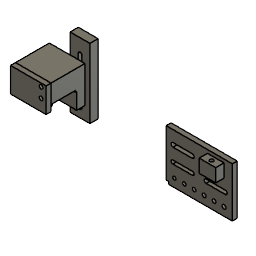
R2_关键配合小样 (Autodesk Fusion 360 design; units mm, degrees)
part number: 2026-09-10-23-08-55-892
part number: 2026-09-10-23-27-46-546
part number: 2026-09-10-23-27-47-376
part number: 2026-09-10-23-27-47-996
part number: 2026-09-10-23-27-48-831
Autodesk Fusion 360 part; units mm, degrees
ref_plane "工作平面1" through (0, 0, 0) normal (0, 0, 1) x (1, 0, 0) in component "CT01_右后承托局部小样"
sketch "草图1" plane through (0, 0, 0) normal (0, 0, 1) x (1, 0, 0) in component "CT01_右后承托局部小样"
  line L0 (-37, 26) -> (6, 26)
  line L1 (6, 26) -> (6, 70)
  line L2 (6, 70) -> (-37, 70)
  line L3 (-37, 70) -> (-37, 26)
  point P0 (-1000, -1000)
  dimension "d14" = 963
  dimension "d15" = 1026
  dimension "d16" = 43
  dimension "d17" = 44
  constraint horizontal L0
  constraint vertical L1
  constraint horizontal L2
  constraint vertical L3
  measures "d14" horizontal distance of L0.start P0
  measures "d15" vertical distance of L0.start P0
  measures "d16" horizontal distance of L0.start L0.end
  measures "d17" vertical distance of L0.end L1.end
extrude "Support_base" add sketch "草图1" along normal blind 10 makes body 1 in component "CT01_右后承托局部小样"
ref_plane "工作平面2" through (0, 0, 10) normal (0, 0, 1) x (1, 0, 0) in component "CT01_右后承托局部小样"
sketch "草图2" plane through (0, 0, 10) normal (0, 0, 1) x (1, 0, 0) in component "CT01_右后承托局部小样"
  line L0 (-37, 47.5) -> (6, 47.5)
  line L1 (6, 47.5) -> (6, 70)
  line L2 (6, 70) -> (-37, 70)
  line L3 (-37, 70) -> (-37, 47.5)
  point P0 (-1000, -1000)
  dimension "d22" = 963
  dimension "d23" = 1047.5
  dimension "d24" = 43
  dimension "d25" = 22.5
  constraint horizontal L0
  constraint vertical L1
  constraint horizontal L2
  constraint vertical L3
  measures "d22" horizontal distance of L0.start P0
  measures "d23" vertical distance of L0.start P0
  measures "d24" horizontal distance of L0.start L0.end
  measures "d25" vertical distance of L0.end L1.end
extrude "Hard_standoff" add sketch "草图2" along normal blind 31 bodies 1 in component "CT01_右后承托局部小样"
ref_plane "工作平面3" through (0, 0, 10) normal (0, 0, 1) x (1, 0, 0) in component "CT01_右后承托局部小样"
sketch "草图3" plane through (0, 0, 10) normal (0, 0, 1) x (1, 0, 0) in component "CT01_右后承托局部小样"
  line L0 (-37, 45.5) -> (6, 45.5)
  line L1 (6, 45.5) -> (6, 47.5)
  line L2 (6, 47.5) -> (-37, 47.5)
  line L3 (-37, 47.5) -> (-37, 45.5)
  point P0 (-1000, -1000)
  dimension "d30" = 963
  dimension "d31" = 1045.5
  dimension "d32" = 43
  dimension "d33" = 2
  constraint horizontal L0
  constraint vertical L1
  constraint horizontal L2
  constraint vertical L3
  measures "d30" horizontal distance of L0.start P0
  measures "d31" vertical distance of L0.start P0
  measures "d32" horizontal distance of L0.start L0.end
  measures "d33" vertical distance of L0.end L1.end
extrude "Lower_Y_stop" add sketch "草图3" along normal blind 1.5 bodies 1 in component "CT01_右后承托局部小样"
ref_plane "工作平面4" through (0, 0, 39.5) normal (0, 0, 1) x (1, 0, 0) in component "CT01_右后承托局部小样"
sketch "草图4" plane through (0, 0, 39.5) normal (0, 0, 1) x (1, 0, 0) in component "CT01_右后承托局部小样"
  line L0 (-37, 45.5) -> (6, 45.5)
  line L1 (6, 45.5) -> (6, 47.5)
  line L2 (6, 47.5) -> (-37, 47.5)
  line L3 (-37, 47.5) -> (-37, 45.5)
  point P0 (-1000, -1000)
  dimension "d38" = 963
  dimension "d39" = 1045.5
  dimension "d40" = 43
  dimension "d41" = 2
  constraint horizontal L0
  constraint vertical L1
  constraint horizontal L2
  constraint vertical L3
  measures "d38" horizontal distance of L0.start P0
  measures "d39" vertical distance of L0.start P0
  measures "d40" horizontal distance of L0.start L0.end
  measures "d41" vertical distance of L0.end L1.end
extrude "Upper_Y_stop" add sketch "草图4" along normal blind 1.5 bodies 1 in component "CT01_右后承托局部小样"
ref_plane "工作平面5" through (0, 0, -1) normal (0, 0, 1) x (1, 0, 0) in component "CT01_右后承托局部小样"
sketch "草图5" plane through (0, 0, -1) normal (0, 0, 1) x (1, 0, 0) in component "CT01_右后承托局部小样"
  circle A0 centre (0, 54) radius 2.25
  point P0 (-1000, -1000)
  dimension "d46" = 1000
  dimension "d47" = 1054
  dimension "d48" = 4.5
  measures "d46" horizontal distance of A0.centre P0
  measures "d47" vertical distance of A0.centre P0
  measures "d48" diameter of A0
extrude "Two_through_bolts_1" cut sketch "草图5" along normal blind 43 bodies 1 in component "CT01_右后承托局部小样"
ref_plane "工作平面6" through (0, 0, -1) normal (0, 0, 1) x (1, 0, 0) in component "CT01_右后承托局部小样"
sketch "草图6" plane through (0, 0, -1) normal (0, 0, 1) x (1, 0, 0) in component "CT01_右后承托局部小样"
  circle A0 centre (0, 66) radius 2.25
  point P0 (-1000, -1000)
  dimension "d53" = 1000
  dimension "d54" = 1066
  dimension "d55" = 4.5
  measures "d53" horizontal distance of A0.centre P0
  measures "d54" vertical distance of A0.centre P0
  measures "d55" diameter of A0
extrude "Two_through_bolts_2" cut sketch "草图6" along normal blind 43 bodies 1 in component "CT01_右后承托局部小样"
ref_plane "工作平面1" through (0, 0, 41) normal (0, 0, 1) x (1, 0, 0) in component "CT02_右后防脱及X止挡局部小样"
sketch "草图1 (2)" plane through (0, 0, 41) normal (0, 0, 1) x (1, 0, 0) in component "CT02_右后防脱及X止挡局部小样"
  line L0 (-37, 40) -> (6, 40)
  line L1 (6, 40) -> (6, 70)
  line L2 (6, 70) -> (-37, 70)
  line L3 (-37, 70) -> (-37, 40)
  point P0 (-1000, -1000)
  dimension "d60" = 963
  dimension "d61" = 1040
  dimension "d62" = 43
  dimension "d63" = 30
  constraint horizontal L0
  constraint vertical L1
  constraint horizontal L2
  constraint vertical L3
  measures "d60" horizontal distance of L0.start P0
  measures "d61" vertical distance of L0.start P0
  measures "d62" horizontal distance of L0.start L0.end
  measures "d63" vertical distance of L0.end L1.end
extrude "Retainer" add sketch "草图1 (2)" along normal blind 6 separate body makes body 2 in component "CT02_右后防脱及X止挡局部小样"
ref_plane "工作平面2" through (0, 0, 39.5) normal (0, 0, 1) x (1, 0, 0) in component "CT02_右后防脱及X止挡局部小样"
sketch "草图2 (2)" plane through (0, 0, 39.5) normal (0, 0, 1) x (1, 0, 0) in component "CT02_右后防脱及X止挡局部小样"
  line L0 (-19.5, 40) -> (-15.5, 40)
  line L1 (-15.5, 40) -> (-15.5, 44.75)
  line L2 (-15.5, 44.75) -> (-19.5, 44.75)
  line L3 (-19.5, 44.75) -> (-19.5, 40)
  point P0 (-1000, -1000)
  dimension "d68" = 980.5
  dimension "d69" = 1040
  dimension "d70" = 4
  dimension "d71" = 4.75
  constraint horizontal L0
  constraint vertical L1
  constraint horizontal L2
  constraint vertical L3
  measures "d68" horizontal distance of L0.start P0
  measures "d69" vertical distance of L0.start P0
  measures "d70" horizontal distance of L0.start L0.end
  measures "d71" vertical distance of L0.end L1.end
extrude "Upper_X_stop" add sketch "草图2 (2)" along normal blind 1.5 bodies 2 in component "CT02_右后防脱及X止挡局部小样"
ref_plane "工作平面3" through (0, 0, 40) normal (0, 0, 1) x (1, 0, 0) in component "CT02_右后防脱及X止挡局部小样"
sketch "草图3 (2)" plane through (0, 0, 40) normal (0, 0, 1) x (1, 0, 0) in component "CT02_右后防脱及X止挡局部小样"
  circle A0 centre (0, 54) radius 2.25
  point P0 (-1000, -1000)
  dimension "d76" = 1000
  dimension "d77" = 1054
  dimension "d78" = 4.5
  measures "d76" horizontal distance of A0.centre P0
  measures "d77" vertical distance of A0.centre P0
  measures "d78" diameter of A0
extrude "Two_through_bolts_1'" cut sketch "草图3 (2)" along normal blind 8 bodies 2 in component "CT02_右后防脱及X止挡局部小样"
ref_plane "工作平面4" through (0, 0, 40) normal (0, 0, 1) x (1, 0, 0) in component "CT02_右后防脱及X止挡局部小样"
sketch "草图4 (2)" plane through (0, 0, 40) normal (0, 0, 1) x (1, 0, 0) in component "CT02_右后防脱及X止挡局部小样"
  circle A0 centre (0, 66) radius 2.25
  point P0 (-1000, -1000)
  dimension "d83" = 1000
  dimension "d84" = 1066
  dimension "d85" = 4.5
  measures "d83" horizontal distance of A0.centre P0
  measures "d84" vertical distance of A0.centre P0
  measures "d85" diameter of A0
extrude "Two_through_bolts_2'" cut sketch "草图4 (2)" along normal blind 8 bodies 2 in component "CT02_右后防脱及X止挡局部小样"
ref_plane "工作平面1" through (0, 0, -10) normal (0, 0, 1) x (1, 0, 0) in component "CT03_托臂槽段试装垫座"
sketch "草图1 (3)" plane through (0, 0, -10) normal (0, 0, 1) x (1, 0, 0) in component "CT03_托臂槽段试装垫座"
  line L0 (-12, 10) -> (12, 10)
  line L1 (12, 10) -> (12, 94)
  line L2 (12, 94) -> (-12, 94)
  line L3 (-12, 94) -> (-12, 10)
  point P0 (-1000, -1000)
  dimension "d90" = 988
  dimension "d91" = 1010
  dimension "d92" = 24
  dimension "d93" = 84
  constraint horizontal L0
  constraint vertical L1
  constraint horizontal L2
  constraint vertical L3
  measures "d90" horizontal distance of L0.start P0
  measures "d91" vertical distance of L0.start P0
  measures "d92" horizontal distance of L0.start L0.end
  measures "d93" vertical distance of L0.end L1.end
extrude "Arm_segment" add sketch "草图1 (3)" along normal blind 10 separate body makes body 3 in component "CT03_托臂槽段试装垫座"
ref_plane "工作平面2" through (0, 0, -11) normal (0, 0, 1) x (1, 0, 0) in component "CT03_托臂槽段试装垫座"
sketch "草图2 (3)" plane through (0, 0, -11) normal (0, 0, 1) x (1, 0, 0) in component "CT03_托臂槽段试装垫座"
  line L0 (-2.25, 21.25) -> (2.25, 21.25)
  line L1 (2.25, 21.25) -> (2.25, 76.75)
  line L2 (2.25, 76.75) -> (-2.25, 76.75)
  line L3 (-2.25, 76.75) -> (-2.25, 21.25)
  point P0 (-1000, -1000)
  dimension "d98" = 997.75
  dimension "d99" = 1021.25
  dimension "d100" = 4.5
  dimension "d101" = 55.5
  constraint horizontal L0
  constraint vertical L1
  constraint horizontal L2
  constraint vertical L3
  measures "d98" horizontal distance of L0.start P0
  measures "d99" vertical distance of L0.start P0
  measures "d100" horizontal distance of L0.start L0.end
  measures "d101" vertical distance of L0.end L1.end
extrude "Pad_mount_slot_0_middle" cut sketch "草图2 (3)" along normal blind 12 bodies 3 in component "CT03_托臂槽段试装垫座"
ref_plane "工作平面3" through (0, 0, -11) normal (0, 0, 1) x (1, 0, 0) in component "CT03_托臂槽段试装垫座"
sketch "草图3 (3)" plane through (0, 0, -11) normal (0, 0, 1) x (1, 0, 0) in component "CT03_托臂槽段试装垫座"
  circle A0 centre (0, 21.25) radius 2.25
  point P0 (-1000, -1000)
  dimension "d106" = 1000
  dimension "d107" = 1021.25
  dimension "d108" = 4.5
  measures "d106" horizontal distance of A0.centre P0
  measures "d107" vertical distance of A0.centre P0
  measures "d108" diameter of A0
extrude "Pad_mount_slot_0_ends_1" cut sketch "草图3 (3)" along normal blind 12 bodies 3 in component "CT03_托臂槽段试装垫座"
ref_plane "工作平面4" through (0, 0, -11) normal (0, 0, 1) x (1, 0, 0) in component "CT03_托臂槽段试装垫座"
sketch "草图4 (3)" plane through (0, 0, -11) normal (0, 0, 1) x (1, 0, 0) in component "CT03_托臂槽段试装垫座"
  circle A0 centre (0, 76.75) radius 2.25
  point P0 (-1000, -1000)
  dimension "d113" = 1000
  dimension "d114" = 1076.75
  dimension "d115" = 4.5
  measures "d113" horizontal distance of A0.centre P0
  measures "d114" vertical distance of A0.centre P0
  measures "d115" diameter of A0
extrude "Pad_mount_slot_0_ends_2" cut sketch "草图4 (3)" along normal blind 12 bodies 3 in component "CT03_托臂槽段试装垫座"
ref_plane "工作平面1" through (0, 0, 0) normal (0, 0, 1) x (1, 0, 0) in component "HT01_孔槽及横孔试片"
sketch "草图1 (4)" plane through (0, 0, 0) normal (0, 0, 1) x (1, 0, 0) in component "HT01_孔槽及横孔试片"
  line L0 (0, 0) -> (80, 0)
  line L1 (80, 0) -> (80, 60)
  line L2 (80, 60) -> (0, 60)
  line L3 (0, 60) -> (0, 0)
  point P0 (-1000, -1000)
  dimension "d120" = 1000
  dimension "d121" = 1000
  dimension "d122" = 80
  dimension "d123" = 60
  constraint horizontal L0
  constraint vertical L1
  constraint horizontal L2
  constraint vertical L3
  measures "d120" horizontal distance of L0.start P0
  measures "d121" vertical distance of L0.start P0
  measures "d122" horizontal distance of L0.start L0.end
  measures "d123" vertical distance of L0.end L1.end
extrude "Base" add sketch "草图1 (4)" along normal blind 6 separate body makes body 4 in component "HT01_孔槽及横孔试片"
ref_plane "工作平面2" through (0, 0, -1) normal (0, 0, 1) x (1, 0, 0) in component "HT01_孔槽及横孔试片"
sketch "草图2 (4)" plane through (0, 0, -1) normal (0, 0, 1) x (1, 0, 0) in component "HT01_孔槽及横孔试片"
  circle A0 centre (10, 10) radius 2
  point P0 (-1000, -1000)
  dimension "d128" = 1010
  dimension "d129" = 1010
  dimension "d130" = 4
  measures "d128" horizontal distance of A0.centre P0
  measures "d129" vertical distance of A0.centre P0
  measures "d130" diameter of A0
extrude "Vertical_4_1" cut sketch "草图2 (4)" along normal blind 8 bodies 4 in component "HT01_孔槽及横孔试片"
ref_plane "工作平面3" through (0, 0, -1) normal (0, 0, 1) x (1, 0, 0) in component "HT01_孔槽及横孔试片"
sketch "草图3 (4)" plane through (0, 0, -1) normal (0, 0, 1) x (1, 0, 0) in component "HT01_孔槽及横孔试片"
  circle A0 centre (22, 10) radius 2.1
  point P0 (-1000, -1000)
  dimension "d135" = 1022
  dimension "d136" = 1010
  dimension "d137" = 4.2
  measures "d135" horizontal distance of A0.centre P0
  measures "d136" vertical distance of A0.centre P0
  measures "d137" diameter of A0
extrude "Vertical_4.2_1" cut sketch "草图3 (4)" along normal blind 8 bodies 4 in component "HT01_孔槽及横孔试片"
ref_plane "工作平面4" through (0, 0, -1) normal (0, 0, 1) x (1, 0, 0) in component "HT01_孔槽及横孔试片"
sketch "草图4 (4)" plane through (0, 0, -1) normal (0, 0, 1) x (1, 0, 0) in component "HT01_孔槽及横孔试片"
  circle A0 centre (34, 10) radius 2.2
  point P0 (-1000, -1000)
  dimension "d142" = 1034
  dimension "d143" = 1010
  dimension "d144" = 4.4
  measures "d142" horizontal distance of A0.centre P0
  measures "d143" vertical distance of A0.centre P0
  measures "d144" diameter of A0
extrude "Vertical_4.4_1" cut sketch "草图4 (4)" along normal blind 8 bodies 4 in component "HT01_孔槽及横孔试片"
ref_plane "工作平面5" through (0, 0, -1) normal (0, 0, 1) x (1, 0, 0) in component "HT01_孔槽及横孔试片"
sketch "草图5 (2)" plane through (0, 0, -1) normal (0, 0, 1) x (1, 0, 0) in component "HT01_孔槽及横孔试片"
  circle A0 centre (46, 10) radius 2.25
  point P0 (-1000, -1000)
  dimension "d149" = 1046
  dimension "d150" = 1010
  dimension "d151" = 4.5
  measures "d149" horizontal distance of A0.centre P0
  measures "d150" vertical distance of A0.centre P0
  measures "d151" diameter of A0
extrude "Vertical_4.5_1" cut sketch "草图5 (2)" along normal blind 8 bodies 4 in component "HT01_孔槽及横孔试片"
ref_plane "工作平面6" through (0, 0, -1) normal (0, 0, 1) x (1, 0, 0) in component "HT01_孔槽及横孔试片"
sketch "草图6 (2)" plane through (0, 0, -1) normal (0, 0, 1) x (1, 0, 0) in component "HT01_孔槽及横孔试片"
  circle A0 centre (58, 10) radius 2.3
  point P0 (-1000, -1000)
  dimension "d156" = 1058
  dimension "d157" = 1010
  dimension "d158" = 4.6
  measures "d156" horizontal distance of A0.centre P0
  measures "d157" vertical distance of A0.centre P0
  measures "d158" diameter of A0
extrude "Vertical_4.6_1" cut sketch "草图6 (2)" along normal blind 8 bodies 4 in component "HT01_孔槽及横孔试片"
ref_plane "工作平面7" through (0, 0, -1) normal (0, 0, 1) x (1, 0, 0) in component "HT01_孔槽及横孔试片"
sketch "草图7" plane through (0, 0, -1) normal (0, 0, 1) x (1, 0, 0) in component "HT01_孔槽及横孔试片"
  circle A0 centre (70, 10) radius 2.4
  point P0 (-1000, -1000)
  dimension "d163" = 1070
  dimension "d164" = 1010
  dimension "d165" = 4.8
  measures "d163" horizontal distance of A0.centre P0
  measures "d164" vertical distance of A0.centre P0
  measures "d165" diameter of A0
extrude "Vertical_4.8_1" cut sketch "草图7" along normal blind 8 bodies 4 in component "HT01_孔槽及横孔试片"
ref_plane "工作平面8" through (0, 0, -1) normal (0, 0, 1) x (1, 0, 0) in component "HT01_孔槽及横孔试片"
sketch "草图8" plane through (0, 0, -1) normal (0, 0, 1) x (1, 0, 0) in component "HT01_孔槽及横孔试片"
  line L0 (8.1, 23.9) -> (31.9, 23.9)
  line L1 (31.9, 23.9) -> (31.9, 28.1)
  line L2 (31.9, 28.1) -> (8.1, 28.1)
  line L3 (8.1, 28.1) -> (8.1, 23.9)
  point P0 (-1000, -1000)
  dimension "d170" = 1008.1
  dimension "d171" = 1023.9
  dimension "d172" = 23.8
  dimension "d173" = 4.2
  constraint horizontal L0
  constraint vertical L1
  constraint horizontal L2
  constraint vertical L3
  measures "d170" horizontal distance of L0.start P0
  measures "d171" vertical distance of L0.start P0
  measures "d172" horizontal distance of L0.start L0.end
  measures "d173" vertical distance of L0.end L1.end
extrude "Slot_4.2_0_middle" cut sketch "草图8" along normal blind 8 bodies 4 in component "HT01_孔槽及横孔试片"
ref_plane "工作平面9" through (0, 0, -1) normal (0, 0, 1) x (1, 0, 0) in component "HT01_孔槽及横孔试片"
sketch "草图9" plane through (0, 0, -1) normal (0, 0, 1) x (1, 0, 0) in component "HT01_孔槽及横孔试片"
  circle A0 centre (8.1, 26) radius 2.1
  point P0 (-1000, -1000)
  dimension "d178" = 1008.1
  dimension "d179" = 1026
  dimension "d180" = 4.2
  measures "d178" horizontal distance of A0.centre P0
  measures "d179" vertical distance of A0.centre P0
  measures "d180" diameter of A0
extrude "Slot_4.2_0_ends_1" cut sketch "草图9" along normal blind 8 bodies 4 in component "HT01_孔槽及横孔试片"
ref_plane "工作平面10" through (0, 0, -1) normal (0, 0, 1) x (1, 0, 0) in component "HT01_孔槽及横孔试片"
sketch "草图10" plane through (0, 0, -1) normal (0, 0, 1) x (1, 0, 0) in component "HT01_孔槽及横孔试片"
  circle A0 centre (31.9, 26) radius 2.1
  point P0 (-1000, -1000)
  dimension "d185" = 1031.9
  dimension "d186" = 1026
  dimension "d187" = 4.2
  measures "d185" horizontal distance of A0.centre P0
  measures "d186" vertical distance of A0.centre P0
  measures "d187" diameter of A0
extrude "Slot_4.2_0_ends_2" cut sketch "草图10" along normal blind 8 bodies 4 in component "HT01_孔槽及横孔试片"
ref_plane "工作平面11" through (0, 0, -1) normal (0, 0, 1) x (1, 0, 0) in component "HT01_孔槽及横孔试片"
sketch "草图11" plane through (0, 0, -1) normal (0, 0, 1) x (1, 0, 0) in component "HT01_孔槽及横孔试片"
  line L0 (48.25, 23.75) -> (71.75, 23.75)
  line L1 (71.75, 23.75) -> (71.75, 28.25)
  line L2 (71.75, 28.25) -> (48.25, 28.25)
  line L3 (48.25, 28.25) -> (48.25, 23.75)
  point P0 (-1000, -1000)
  dimension "d192" = 1048.25
  dimension "d193" = 1023.75
  dimension "d194" = 23.5
  dimension "d195" = 4.5
  constraint horizontal L0
  constraint vertical L1
  constraint horizontal L2
  constraint vertical L3
  measures "d192" horizontal distance of L0.start P0
  measures "d193" vertical distance of L0.start P0
  measures "d194" horizontal distance of L0.start L0.end
  measures "d195" vertical distance of L0.end L1.end
extrude "Slot_4.5_0_middle" cut sketch "草图11" along normal blind 8 bodies 4 in component "HT01_孔槽及横孔试片"
ref_plane "工作平面12" through (0, 0, -1) normal (0, 0, 1) x (1, 0, 0) in component "HT01_孔槽及横孔试片"
sketch "草图12" plane through (0, 0, -1) normal (0, 0, 1) x (1, 0, 0) in component "HT01_孔槽及横孔试片"
  circle A0 centre (48.25, 26) radius 2.25
  point P0 (-1000, -1000)
  dimension "d200" = 1048.25
  dimension "d201" = 1026
  dimension "d202" = 4.5
  measures "d200" horizontal distance of A0.centre P0
  measures "d201" vertical distance of A0.centre P0
  measures "d202" diameter of A0
extrude "Slot_4.5_0_ends_1" cut sketch "草图12" along normal blind 8 bodies 4 in component "HT01_孔槽及横孔试片"
ref_plane "工作平面13" through (0, 0, -1) normal (0, 0, 1) x (1, 0, 0) in component "HT01_孔槽及横孔试片"
sketch "草图13" plane through (0, 0, -1) normal (0, 0, 1) x (1, 0, 0) in component "HT01_孔槽及横孔试片"
  circle A0 centre (71.75, 26) radius 2.25
  point P0 (-1000, -1000)
  dimension "d207" = 1071.75
  dimension "d208" = 1026
  dimension "d209" = 4.5
  measures "d207" horizontal distance of A0.centre P0
  measures "d208" vertical distance of A0.centre P0
  measures "d209" diameter of A0
extrude "Slot_4.5_0_ends_2" cut sketch "草图13" along normal blind 8 bodies 4 in component "HT01_孔槽及横孔试片"
ref_plane "工作平面14" through (0, 0, -1) normal (0, 0, 1) x (1, 0, 0) in component "HT01_孔槽及横孔试片"
sketch "草图14" plane through (0, 0, -1) normal (0, 0, 1) x (1, 0, 0) in component "HT01_孔槽及横孔试片"
  line L0 (8.4, 41.6) -> (31.6, 41.6)
  line L1 (31.6, 41.6) -> (31.6, 46.4)
  line L2 (31.6, 46.4) -> (8.4, 46.4)
  line L3 (8.4, 46.4) -> (8.4, 41.6)
  point P0 (-1000, -1000)
  dimension "d214" = 1008.4
  dimension "d215" = 1041.6
  dimension "d216" = 23.2
  dimension "d217" = 4.8
  constraint horizontal L0
  constraint vertical L1
  constraint horizontal L2
  constraint vertical L3
  measures "d214" horizontal distance of L0.start P0
  measures "d215" vertical distance of L0.start P0
  measures "d216" horizontal distance of L0.start L0.end
  measures "d217" vertical distance of L0.end L1.end
extrude "Slot_4.8_0_middle" cut sketch "草图14" along normal blind 8 bodies 4 in component "HT01_孔槽及横孔试片"
ref_plane "工作平面15" through (0, 0, -1) normal (0, 0, 1) x (1, 0, 0) in component "HT01_孔槽及横孔试片"
sketch "草图15" plane through (0, 0, -1) normal (0, 0, 1) x (1, 0, 0) in component "HT01_孔槽及横孔试片"
  circle A0 centre (8.4, 44) radius 2.4
  point P0 (-1000, -1000)
  dimension "d222" = 1008.4
  dimension "d223" = 1044
  dimension "d224" = 4.8
  measures "d222" horizontal distance of A0.centre P0
  measures "d223" vertical distance of A0.centre P0
  measures "d224" diameter of A0
extrude "Slot_4.8_0_ends_1" cut sketch "草图15" along normal blind 8 bodies 4 in component "HT01_孔槽及横孔试片"
ref_plane "工作平面16" through (0, 0, -1) normal (0, 0, 1) x (1, 0, 0) in component "HT01_孔槽及横孔试片"
sketch "草图16" plane through (0, 0, -1) normal (0, 0, 1) x (1, 0, 0) in component "HT01_孔槽及横孔试片"
  circle A0 centre (31.6, 44) radius 2.4
  point P0 (-1000, -1000)
  dimension "d229" = 1031.6
  dimension "d230" = 1044
  dimension "d231" = 4.8
  measures "d229" horizontal distance of A0.centre P0
  measures "d230" vertical distance of A0.centre P0
  measures "d231" diameter of A0
extrude "Slot_4.8_0_ends_2" cut sketch "草图16" along normal blind 8 bodies 4 in component "HT01_孔槽及横孔试片"
ref_plane "工作平面17" through (0, 0, 6) normal (0, 0, 1) x (1, 0, 0) in component "HT01_孔槽及横孔试片"
sketch "草图17" plane through (0, 0, 6) normal (0, 0, 1) x (1, 0, 0) in component "HT01_孔槽及横孔试片"
  line L0 (50, 40) -> (70, 40)
  line L1 (70, 40) -> (70, 56)
  line L2 (70, 56) -> (50, 56)
  line L3 (50, 56) -> (50, 40)
  point P0 (-1000, -1000)
  dimension "d236" = 1050
  dimension "d237" = 1040
  dimension "d238" = 20
  dimension "d239" = 16
  constraint horizontal L0
  constraint vertical L1
  constraint horizontal L2
  constraint vertical L3
  measures "d236" horizontal distance of L0.start P0
  measures "d237" vertical distance of L0.start P0
  measures "d238" horizontal distance of L0.start L0.end
  measures "d239" vertical distance of L0.end L1.end
extrude "Horizontal_hole_boss" add sketch "草图17" along normal blind 10 bodies 4 in component "HT01_孔槽及横孔试片"
ref_plane "工作平面18" through (0, 39, 0) normal (0, 1, 0) x (0, 0, 1) in component "HT01_孔槽及横孔试片"
sketch "草图18" plane through (0, 39, 0) normal (0, 1, 0) x (1, 0, 0) in component "HT01_孔槽及横孔试片"
  circle A0 centre (60, -11) radius 2.25
  point P0 (-1000, -1000)
  dimension "d244" = 1060
  dimension "d245" = 989
  dimension "d246" = 4.5
  measures "d244" horizontal distance of A0.centre P0
  measures "d245" vertical distance of A0.centre P0
  measures "d246" diameter of A0
extrude "Horizontal_M4_1" cut sketch "草图18" along normal blind 18 bodies 4 in component "HT01_孔槽及横孔试片"
ref_plane "工作平面19" through (0, 0, -1) normal (0, 0, 1) x (1, 0, 0) in component "HT01_孔槽及横孔试片"
sketch "草图19" plane through (0, 0, -1) normal (0, 0, 1) x (1, 0, 0) in component "HT01_孔槽及横孔试片"
  line L0 (0, 0) -> (3, 0)
  line L1 (3, 0) -> (3, 3)
  line L2 (3, 3) -> (0, 3)
  line L3 (0, 3) -> (0, 0)
  point P0 (-1000, -1000)
  dimension "d251" = 1000
  dimension "d252" = 1000
  dimension "d253" = 3
  dimension "d254" = 3
  constraint horizontal L0
  constraint vertical L1
  constraint horizontal L2
  constraint vertical L3
  measures "d251" horizontal distance of L0.start P0
  measures "d252" vertical distance of L0.start P0
  measures "d253" horizontal distance of L0.start L0.end
  measures "d254" vertical distance of L0.end L1.end
extrude "Origin_notch" cut sketch "草图19" along normal blind 8 bodies 4 in component "HT01_孔槽及横孔试片"
component "CT01_右后承托局部小样" placed x (1, 0, 0) y (0, 1, 0) z (0, 0, 1) at (0, 0, 0)
component "CT02_右后防脱及X止挡局部小样" placed x (1, 0, 0) y (0, 1, 0) z (0, 0, 1) at (0, 0, 0)
component "CT03_托臂槽段试装垫座" placed x (1, 0, 0) y (0, 1, 0) z (0, 0, 1) at (0, 0, 0)
component "HT01_孔槽及横孔试片" placed x (1, 0, 0) y (0, 1, 0) z (0, 0, 1) at (110, 0, 0)
equation "pad_w = 74 mm" comment "TEST_COUPON_ASSUMED_VERIFY_WITH_REAL_PARTS"
equation "coupon_w = 43 mm" comment "TEST_COUPON_ASSUMED_VERIFY_WITH_REAL_PARTS"
equation "board_w = 90 mm" comment "TEST_COUPON_ASSUMED_VERIFY_WITH_REAL_PARTS"
equation "pad_t = 10 mm" comment "TEST_COUPON_ASSUMED_VERIFY_WITH_REAL_PARTS"
equation "soft_t = 0.5 mm" comment "TEST_COUPON_ASSUMED_VERIFY_WITH_REAL_PARTS"
equation "stack_h = 30 mm" comment "TEST_COUPON_ASSUMED_VERIFY_WITH_REAL_PARTS"
equation "retainer_gap = 0.5 mm" comment "TEST_COUPON_ASSUMED_VERIFY_WITH_REAL_PARTS"
equation "lateral_gap = 1 mm" comment "TEST_COUPON_ASSUMED_VERIFY_WITH_REAL_PARTS"
equation "acrylic_t = 1 mm" comment "TEST_COUPON_ASSUMED_VERIFY_WITH_REAL_PARTS"
equation "slot_d = 4.5 mm" comment "TEST_COUPON_ASSUMED_VERIFY_WITH_REAL_PARTS"
equation "support_depth = 19 mm" comment "TEST_COUPON_ASSUMED_VERIFY_WITH_REAL_PARTS"
equation "d14 = 1000 mm + ( -pad_w / 2 )"
equation "d15 = 1000 mm + ( board_w / 2 - support_depth )"
equation "d16 = coupon_w"
equation "d18 = pad_t"
equation "d20 = pad_t"
equation "d22 = 1000 mm + ( -pad_w / 2 )"
equation "d23 = 1000 mm + ( board_w / 2 + lateral_gap / 2 + 2 mm )"
equation "d24 = coupon_w"
equation "d25 = 25 mm - lateral_gap / 2 - 2 mm"
equation "d26 = soft_t + stack_h + retainer_gap"
equation "d28 = pad_t"
equation "d30 = 1000 mm + ( -pad_w / 2 )"
equation "d31 = 1000 mm + ( board_w / 2 + lateral_gap / 2 )"
equation "d32 = coupon_w"
equation "d34 = soft_t + acrylic_t"
equation "d36 = pad_t + soft_t + stack_h - acrylic_t"
equation "d38 = 1000 mm + ( -pad_w / 2 )"
equation "d39 = 1000 mm + ( board_w / 2 + lateral_gap / 2 )"
equation "d40 = coupon_w"
equation "d42 = acrylic_t + retainer_gap"
equation "d46 = 1000 mm + ( 0 mm )"
equation "d47 = 1000 mm + ( 54 mm )"
equation "d48 = slot_d"
equation "d49 = pad_t + soft_t + stack_h + retainer_gap + 2 mm"
equation "d53 = 1000 mm + ( 0 mm )"
equation "d54 = 1000 mm + ( 66 mm )"
equation "d55 = slot_d"
equation "d56 = pad_t + soft_t + stack_h + retainer_gap + 2 mm"
equation "d58 = pad_t + soft_t + stack_h + retainer_gap"
equation "d60 = 1000 mm + ( -pad_w / 2 )"
equation "d61 = 1000 mm + ( 40 mm )"
equation "d62 = coupon_w"
equation "d66 = pad_t + soft_t + stack_h - acrylic_t"
equation "d68 = 1000 mm + ( -20 mm + lateral_gap / 2 )"
equation "d69 = 1000 mm + ( 40 mm )"
equation "d72 = acrylic_t + retainer_gap"
equation "d74 = pad_t + soft_t + stack_h + retainer_gap - 1 mm"
equation "d76 = 1000 mm + ( 0 mm )"
equation "d77 = 1000 mm + ( 54 mm )"
equation "d78 = slot_d"
equation "d81 = pad_t + soft_t + stack_h + retainer_gap - 1 mm"
equation "d83 = 1000 mm + ( 0 mm )"
equation "d84 = 1000 mm + ( 66 mm )"
equation "d85 = slot_d"
equation "d90 = 1000 mm + ( -12 mm )"
equation "d91 = 1000 mm + ( 10 mm )"
equation "d98 = 1000 mm + ( ( 0 mm ) - ( ( slot_d ) / 2 ) )"
equation "d99 = 1000 mm + ( ( 49 mm ) - ( ( 60 mm - slot_d ) / 2 ) )"
equation "d100 = slot_d"
equation "d101 = 2 * ( ( 60 mm - slot_d ) / 2 )"
equation "d106 = 1000 mm + ( 0 mm )"
equation "d107 = 1000 mm + ( ( 49 mm ) - ( ( 60 mm - slot_d ) / 2 ) )"
equation "d108 = slot_d"
equation "d113 = 1000 mm + ( 0 mm )"
equation "d114 = 1000 mm + ( ( 49 mm ) + ( ( 60 mm - slot_d ) / 2 ) )"
equation "d115 = slot_d"
equation "d120 = 1000 mm + ( 0 mm )"
equation "d121 = 1000 mm + ( 0 mm )"
equation "d128 = 1000 mm + ( 10 mm )"
equation "d129 = 1000 mm + ( 10 mm )"
equation "d135 = 1000 mm + ( 22 mm )"
equation "d136 = 1000 mm + ( 10 mm )"
equation "d142 = 1000 mm + ( 34 mm )"
equation "d143 = 1000 mm + ( 10 mm )"
equation "d149 = 1000 mm + ( 46 mm )"
equation "d150 = 1000 mm + ( 10 mm )"
equation "d156 = 1000 mm + ( 58 mm )"
equation "d157 = 1000 mm + ( 10 mm )"
equation "d163 = 1000 mm + ( 70 mm )"
equation "d164 = 1000 mm + ( 10 mm )"
equation "d170 = 1000 mm + ( ( 20 mm ) - ( ( 28 mm - 4.2 mm ) / 2 ) )"
equation "d171 = 1000 mm + ( ( 26 mm ) - ( ( 4.2 mm ) / 2 ) )"
equation "d172 = 2 * ( ( 28 mm - 4.2 mm ) / 2 )"
equation "d178 = 1000 mm + ( ( 20 mm ) - ( ( 28 mm - 4.2 mm ) / 2 ) )"
equation "d179 = 1000 mm + ( 26 mm )"
equation "d185 = 1000 mm + ( ( 20 mm ) + ( ( 28 mm - 4.2 mm ) / 2 ) )"
equation "d186 = 1000 mm + ( 26 mm )"
equation "d192 = 1000 mm + ( ( 60 mm ) - ( ( 28 mm - 4.5 mm ) / 2 ) )"
equation "d193 = 1000 mm + ( ( 26 mm ) - ( ( 4.5 mm ) / 2 ) )"
equation "d194 = 2 * ( ( 28 mm - 4.5 mm ) / 2 )"
equation "d200 = 1000 mm + ( ( 60 mm ) - ( ( 28 mm - 4.5 mm ) / 2 ) )"
equation "d201 = 1000 mm + ( 26 mm )"
equation "d207 = 1000 mm + ( ( 60 mm ) + ( ( 28 mm - 4.5 mm ) / 2 ) )"
equation "d208 = 1000 mm + ( 26 mm )"
equation "d214 = 1000 mm + ( ( 20 mm ) - ( ( 28 mm - 4.8 mm ) / 2 ) )"
equation "d215 = 1000 mm + ( ( 44 mm ) - ( ( 4.8 mm ) / 2 ) )"
equation "d216 = 2 * ( ( 28 mm - 4.8 mm ) / 2 )"
equation "d222 = 1000 mm + ( ( 20 mm ) - ( ( 28 mm - 4.8 mm ) / 2 ) )"
equation "d223 = 1000 mm + ( 44 mm )"
equation "d229 = 1000 mm + ( ( 20 mm ) + ( ( 28 mm - 4.8 mm ) / 2 ) )"
equation "d230 = 1000 mm + ( 44 mm )"
equation "d236 = 1000 mm + ( 50 mm )"
equation "d237 = 1000 mm + ( 40 mm )"
equation "d244 = 1000 mm + ( 60 mm )"
equation "d245 = 1000 mm + ( -( 11 mm ) )"
equation "d251 = 1000 mm + ( 0 mm )"
equation "d252 = 1000 mm + ( 0 mm )"
